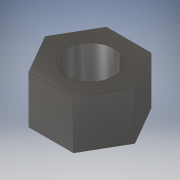
# Autodesk Inventor part: Nut thing
Saved by Autodesk Inventor 2018 (Build 220112000, 112)
## iProperties
Created: 2018-10-23
Part Number: Nut thing
Material: Generic
Document SubType Name: Modeling
Designer: Melda
Density: 1 g/cm^3
Appearance: Knurled 45
Author: Melda
Autodesk Inventor part; units mm, degrees
ref_plane "YZ Plane" through (0, 0, 0) normal (1, 0, 0) x (0, 1, 0)
ref_plane "XZ Plane" through (0, 0, 0) normal (0, 1, 0) x (-1, 0, 0)
ref_plane "XY Plane" through (0, 0, 0) normal (0, 0, 1) x (1, 0, 0)
sketch "Sketch1" plane through (0, 0, 0) normal (0, 1, 0) x (-1, 0, 0)
  circle A0 centre (0, 0) radius 4
  line L0 (7.5, 0) -> (3.75, -6.4952)
  line L1 (3.75, -6.4952) -> (-3.75, -6.4952)
  line L2 (-3.75, -6.4952) -> (-7.5, 0)
  line L3 (-7.5, 0) -> (-3.75, 6.4952)
  line L4 (-3.75, 6.4952) -> (3.75, 6.4952)
  line L5 (3.75, 6.4952) -> (7.5, 0)
  dimension "d0" = 8
  dimension "d1" = 15
  constraints: 12 end point, 2 coincident, 1 centre point, 13 other
  measures "d0" diameter of A0
  measures "d1" distance of L2.end L0.start
extrude "Extrusion1" add sketch "Sketch1" along normal blind 8
body "Solid1"
